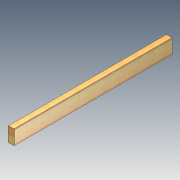
# Autodesk Inventor part: GE-12103-03
Saved by Autodesk Inventor 2012 (Build 160160000, 160)
## iProperties
Created: 2011-11-27
Part Number: GE-12103-03
Document SubType Name: Modeling
Designer: dfoster
Density: 1 g/cm^3
Description: Brace, 2x4
Material: Default
Title: Brace, 2x4
Author: dfoster
Autodesk Inventor part; units mm, degrees
ref_plane "YZ Plane" through (0, 0, 0) normal (1, 0, 0) x (0, 1, 0)
ref_plane "XZ Plane" through (0, 0, 0) normal (0, 1, 0) x (-1, 0, 0)
ref_plane "XY Plane" through (0, 0, 0) normal (0, 0, 1) x (1, 0, 0)
sketch "Sketch1" plane through (0, 0, 0) normal (0, 0, 1) x (1, 0, 0)
  line L0 (3.175, 0) -> (34.925, 0)
  line L1 (38.1, 3.175) -> (38.1, 85.725)
  line L2 (34.925, 88.9) -> (3.175, 88.9)
  line L3 (0, 85.725) -> (0, 3.175)
  arc A0 (3.175, 88.9) -> (0, 85.725) centre (3.175, 85.725) ccw
  arc A1 (0, 3.175) -> (3.175, 0) centre (3.175, 3.175) ccw
  arc A2 (34.925, 0) -> (38.1, 3.175) centre (34.925, 3.175) ccw
  arc A3 (38.1, 85.725) -> (34.925, 88.9) centre (34.925, 85.725) ccw
  point P0 (0, 0)
  point P1 (38.1, 88.9)
  point P2 (0, 88.9)
  dimension "d0" = 88.9
  dimension "d1" = 38.1
  dimension "d2" = 3.175
  constraints: 8 end point, 8 point on circle, 8 tangent, 6 point on line, 4 centre point, 3 equal radius, 2 horizontal, 2 vertical
  measures "d0" distance of point (0, 88.9) point (0, 0)
  measures "d1" distance of point (38.1, 88.9) point (0, 88.9)
  measures "d2" radius of A0
extrude "Extrusion1" add sketch "Sketch1" along normal blind 952.5
body "Solid1"
